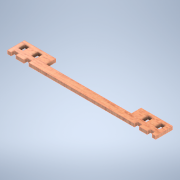
# Autodesk Inventor part: DoorFrameTop_V3
Saved by Autodesk Inventor 2022.2 (Build 262287000, 287)
## iProperties
Created: 2023-03-05
Part Number: DoorFrameTop_V3
Material: Wood (Oak)
Document SubType Name: Modeling
Designer: jaege
Density: 0.76 g/cm^3
Appearance: Red Oak - Natural Low Gloss
Author: jaege
Autodesk Inventor part; units mm, degrees
ref_plane "YZ Plane" through (0, 0, 0) normal (1, 0, 0) x (0, 1, 0)
ref_plane "XZ Plane" through (0, 0, 0) normal (0, 1, 0) x (-1, 0, 0)
ref_plane "XY Plane" through (0, 0, 0) normal (0, 0, 1) x (1, 0, 0)
sketch "Sketch1" plane through (0, 0, 0) normal (0, 1, 0) x (-1, 0, 0)
  line L0 (92, -24.95) -> (53, -24.95)
  line L1 (53, -24.95) -> (53, 0) construction
  line L2 (0, -24.95) -> (0, 0) construction
  line L3 (92, -8) -> (0, -8) construction
  line L4 (92, -4) -> (0, -4) construction
  line L5 (92, -20.95) -> (0, -20.95) construction
  line L6 (53, -24.95) -> (53, -12.9)
  line L7 (92, -12.9) -> (0, -12.9) construction
  line L8 (92, -24.95) -> (0, -24.95) construction
  line L9 (87.5, -24.95) -> (87.5, 0) construction
  line L10 (71.5, -24.95) -> (71.5, 0) construction
  line L11 (65.5, -24.95) -> (65.5, 0) construction
  line L12 (81.5, 0) -> (81.5, -24.95) construction
  line L13 (87.5, -20.95) -> (81.5, -20.95)
  line L14 (81.5, -20.95) -> (81.5, -12.9)
  line L15 (81.5, -12.9) -> (87.5, -12.9)
  line L16 (87.5, -12.9) -> (87.5, -20.95)
  line L17 (71.5, -20.95) -> (65.5, -20.95)
  line L18 (65.5, -20.95) -> (65.5, -12.9)
  line L19 (65.5, -12.9) -> (71.5, -12.9)
  line L20 (71.5, -12.9) -> (71.5, -20.95)
  line L21 (71.5, -8) -> (65.5, -8)
  line L22 (65.5, -8) -> (65.5, -4)
  line L23 (65.5, -4) -> (71.5, -4)
  line L24 (71.5, -4) -> (71.5, -8)
  line L25 (87.5, -8) -> (81.5, -8)
  line L26 (81.5, -8) -> (81.5, -4)
  line L27 (81.5, -4) -> (87.5, -4)
  line L28 (87.5, -4) -> (87.5, -8)
  line L29 (53, -12.9) -> (0, -12.9)
  line L30 (92, 0) -> (0, 0) construction
  line L31 (53, -4) -> (0, -4)
  line L32 (92, -4) -> (87.5, -4)
  line L33 (81.5, -4) -> (71.5, -4)
  line L34 (65.5, -4) -> (53, -4)
  line L35 (92, -24.95) -> (92, 0) construction
  line L36 (92, -24.95) -> (92, -4)
  line L37 (-92, -24.95) -> (-53, -24.95)
  line L38 (-53, -24.95) -> (-53, 0) construction
  line L39 (-92, -8) -> (0, -8) construction
  line L40 (-92, -4) -> (0, -4) construction
  line L41 (-92, -20.95) -> (0, -20.95) construction
  line L42 (-53, -24.95) -> (-53, -12.9)
  line L43 (-92, -12.9) -> (0, -12.9) construction
  line L44 (-92, -24.95) -> (0, -24.95) construction
  line L45 (-87.5, -24.95) -> (-87.5, 0) construction
  line L46 (-71.5, -24.95) -> (-71.5, 0) construction
  line L47 (-65.5, -24.95) -> (-65.5, 0) construction
  line L48 (-81.5, 0) -> (-81.5, -24.95) construction
  line L49 (-87.5, -20.95) -> (-81.5, -20.95)
  line L50 (-81.5, -20.95) -> (-81.5, -12.9)
  line L51 (-81.5, -12.9) -> (-87.5, -12.9)
  line L52 (-87.5, -12.9) -> (-87.5, -20.95)
  line L53 (-71.5, -20.95) -> (-65.5, -20.95)
  line L54 (-65.5, -20.95) -> (-65.5, -12.9)
  line L55 (-65.5, -12.9) -> (-71.5, -12.9)
  line L56 (-71.5, -12.9) -> (-71.5, -20.95)
  line L57 (-71.5, -8) -> (-65.5, -8)
  line L58 (-65.5, -8) -> (-65.5, -4)
  line L59 (-65.5, -4) -> (-71.5, -4)
  line L60 (-71.5, -4) -> (-71.5, -8)
  line L61 (-87.5, -8) -> (-81.5, -8)
  line L62 (-81.5, -8) -> (-81.5, -4)
  line L63 (-81.5, -4) -> (-87.5, -4)
  line L64 (-87.5, -4) -> (-87.5, -8)
  line L65 (-53, -12.9) -> (0, -12.9)
  line L66 (-92, 0) -> (0, 0) construction
  line L67 (-53, -4) -> (0, -4)
  line L68 (-92, -4) -> (-87.5, -4)
  line L69 (-81.5, -4) -> (-71.5, -4)
  line L70 (-65.5, -4) -> (-53, -4)
  line L71 (-92, -24.95) -> (-92, 0) construction
  line L72 (-92, -24.95) -> (-92, -4)
  dimension "d19" = 8.05
  dimension "d20" = 4
  dimension "d21" = 4.9
  dimension "d22" = 4
  dimension "d24" = 6
  dimension "d25" = 10
  dimension "d26" = 6
  dimension "d27" = 12.5
  dimension "d29" = 92
  dimension "d30" = 4
  dimension "d31" = 4.5
  constraints: 147 end point, 51 point on line, 34 symmetric about line, 8 parallel, 7 horizontal, 6 collinear, 6 perpendicular, 2 vertical
  measures "d19" distance between parallel lines of L7 L5
  measures "d20" distance between parallel lines of L8 L5
  measures "d21" distance between parallel lines of L3 L7
  measures "d22" distance between parallel lines of L4 L3
  measures "d24" distance between parallel lines of L12 L9
  measures "d25" distance between parallel lines of L10 L12
  measures "d26" distance between parallel lines of L11 L10
  measures "d27" distance between parallel lines of L6 L11
  measures "d29" distance of L2.start L0.start
  measures "d30" distance between parallel lines of L30 L4
  measures "d31" distance between parallel lines of L9 L35
extrude "Extrusion1" add sketch "Sketch1" along normal blind 4 contours L0 L6 L29 L65 L42 L37 L72 L68 L64 L61 L62 L69 L60 L57 L58 L70 L67 L31 L34 L22 L21 L24 L33 L26 L25 L28 L32 L36
body "Solid1"
